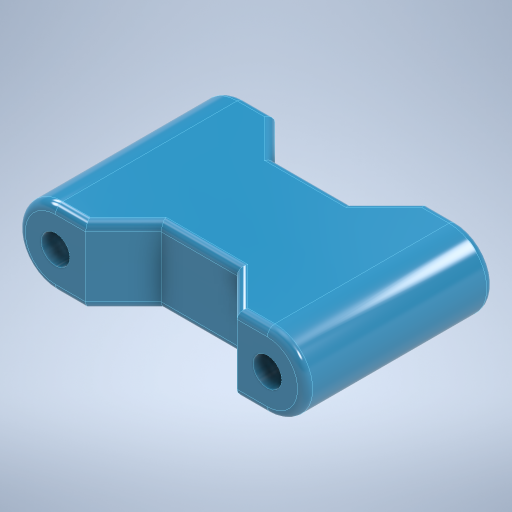
# Autodesk Inventor part: ConectorBrazos
Saved by Autodesk Inventor 2024 (Build 280153000, 153)
## iProperties
Created: 2023-11-02
Part Number: ConectorBrazos
Material: Generic
Document SubType Name: Modeling
Designer: fredy
Density: 1 g/cm^3
Appearance: Sky Blue Dark
Author: fredy
Autodesk Inventor part; units mm, degrees
ref_plane "YZ Plane" through (0, 0, 0) normal (1, 0, 0) x (0, 1, 0)
ref_plane "XZ Plane" through (0, 0, 0) normal (0, 1, 0) x (-1, 0, 0)
ref_plane "XY Plane" through (0, 0, 0) normal (0, 0, 1) x (1, 0, 0)
sketch "Sketch1" plane through (0, 0, 0) normal (0, 0, 1) x (1, 0, 0)
  circle A0 centre (-14, 0) radius 1.8875
  circle A1 centre (-14, 0) radius 5
  line L0 (0, -7) -> (0, 7) projected
  circle A2 centre (14, 0) radius 1.8875
  circle A3 centre (14, 0) radius 5
  line L1 (-14, 5) -> (-5, 5)
  line L2 (-5, 5) -> (0, 5)
  line L3 (14, 5) -> (5, 5)
  line L4 (5, 5) -> (0, 5)
  line L5 (-26.6, 0) -> (26.6, 0) projected
  line L6 (-14, -5) -> (-5, -5)
  line L7 (-5, -5) -> (0, -5)
  line L8 (5, -5) -> (0, -5)
  line L9 (14, -5) -> (5, -5)
  point P0 (0, 0)
  point P1 (14, 5)
  point P2 (-14, -5)
  point P3 (14, -5)
  dimension "d1" = 10
  dimension "d0" = 3.775
  dimension "d2" = 28
  dimension "d3" = 5
  dimension "d4" = 5
  constraints: 16 end point, 9 symmetric about line, 3 centre point, 2 coincident, 1 horizontal, 1 horizontal alignment, 1 perpendicular, 1 point on line, 5 other
  measures "d0" diameter of A0
  measures "d2" distance of A2.centre A0.centre
  measures "d3" distance from line of point (0, 0) L2
  measures "d4" distance of L1.end L2.end
extrude "Extrusion1" add sketch "Sketch1" along normal blind 25 contours L5 A1 A0 | A0 L5 A1 | L5 L0 L7 L6 A1 | A1 L1 L2 L0 L5 | L5 A3 L9 L8 L0 | L0 L4 L3 A3 L5 | L5 A2 A3 | A3 L5 A2
sketch "Sketch2" plane through (-14, 5, 0) normal (0, 1, 0) x (1, 0, 0)
  line L0 (28, -25) -> (0, -25) projected
  line L1 (4, -25) -> (9, -20)
  line L2 (9, -20) -> (14, -20)
  line L3 (28, 0) -> (0, 0) projected
  line L4 (28, 0) -> (28, -25) projected
  line L5 (28, -12.5) -> (1.8875, -12.5)
  line L6 (1.8875, -25) -> (1.8875, 0) projected
  line L7 (28, 0) -> (0, 0)
  line L8 (4, 0) -> (9, -5)
  line L9 (9, -5) -> (14, -5)
  line L10 (14, -25) -> (14, 0)
  line L11 (24, -25) -> (19, -20)
  line L12 (19, -20) -> (14, -20)
  line L13 (24, 0) -> (19, -5)
  line L14 (19, -5) -> (14, -5)
  point P0 (14, 0)
  point P1 (4, 0)
  dimension "d7" = 45
  dimension "d8" = 15
  dimension "d9" = 10
  constraints: 22 end point, 7 symmetric about line, 5 midpoint, 3 point on line, 1 parallel, 1 perpendicular
  measures "d7" angle of L0 L1
  measures "d8" distance of L8.end L1.end
  measures "d9" distance of L11.end L1.end
extrude "Extrusion2" cut sketch "Sketch2" against normal up to surface (10 mm away) contours L0 L10 L12 L11 | L0 L1 L2 L10 | L13 L14 L10 L3 | L9 L8 L3 L10
fillet "Fillet1" radius 1 20 edges at (-12, -5, 25) (-12, 5, 25) (-19, 0, 25) (-7.5, 5, 22.5) (0, 5, 20) (7.5, 5, 22.5) (19, 0, 25) (-7.5, -5, 22.5) (0, -5, 20) (7.5, -5, 22.5) (19, 0, 0) (-12, 5, 0) (-12, -5, 0) (7.5, -5, 2.5) (0, -5, 5) (-7.5, -5, 2.5) (-19, 0, 0) (-7.5, 5, 2.5) (0, 5, 5) (7.5, 5, 2.5)
body "Solid1"
